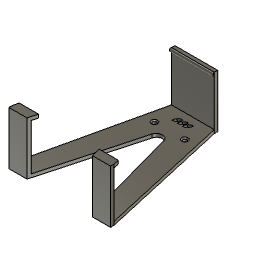
Sega Game Gear (Autodesk Fusion 360 design; units mm, degrees)
Autodesk Fusion 360 part; units mm, degrees
sketch "Top" plane through (0, 0, 0) normal (0, 0, 1) x (1, 0, 0)
  spline S0 degree 3 poles (50.664, -12.787) (49.4535, -14.1293) (47.9947, -14.8503) (47.407, -14.3973) knots 0 0 0 0 1 1 1 1
  spline S1 degree 3 poles (47.407, -14.3973) (46.8193, -13.9442) (47.3242, -12.4896) (48.5334, -11.1472) knots 1 1 1 1 2 2 2 2
  spline S2 degree 3 poles (48.5334, -11.1472) (49.7439, -9.8062) (51.2028, -9.0852) (51.7904, -9.5383) knots 2 2 2 2 3 3 3 3
  spline S3 degree 3 poles (51.7904, -9.5383) (52.3782, -9.9914) (51.8732, -11.446) (50.664, -12.787) knots 3 3 3 3 4 4 4 4
  spline S4 degree 3 poles (42.858, -14.3973) (42.2703, -13.9442) (42.7739, -12.4896) (43.9844, -11.1472) knots 0 0 0 0 1 1 1 1
  spline S5 degree 3 poles (43.9844, -11.1472) (45.1949, -9.8062) (46.6523, -9.0852) (47.2415, -9.5383) knots 1 1 1 1 2 2 2 2
  spline S6 degree 3 poles (47.2415, -9.5383) (47.8292, -9.9914) (47.3242, -11.446) (46.1137, -12.787) knots 2 2 2 2 3 3 3 3
  spline S7 degree 3 poles (46.1137, -12.787) (44.9032, -14.1293) (43.4458, -14.8503) (42.858, -14.3973) knots 3 3 3 3 4 4 4 4
  spline S8 degree 3 poles (38.2038, -14.4127) (37.6302, -13.9568) (38.1225, -12.4924) (39.3008, -11.143) knots 0 0 0 0 1 1 1 1
  spline S9 degree 3 poles (39.3008, -11.143) (40.4791, -9.7922) (41.8986, -9.0684) (42.4723, -9.5229) knots 1 1 1 1 2 2 2 2
  spline S10 degree 3 poles (42.4723, -9.5229) (43.0446, -9.9788) (42.5536, -11.4432) (41.374, -12.7926) knots 2 2 2 2 3 3 3 3
  spline S11 degree 3 poles (41.374, -12.7926) (40.1957, -14.1434) (38.7761, -14.8672) (38.2038, -14.4127) knots 3 3 3 3 4 4 4 4
  line L0 (64, -3) -> (64, 0)
  line L1 (64, 0) -> (26, 0)
  line L2 (26, 0) -> (26, -3)
  line L3 (26, -3) -> (0, -118)
  line L4 (0, -118) -> (0, -121)
  line L5 (0, -121) -> (16, -121)
  line L6 (16, -121) -> (39.812, -33.9631)
  spline S12 degree 3 poles (39.812, -33.9631) (41.2562, -28.684) (48.7438, -28.684) (50.188, -33.9631) knots 7 7 7 7 8 8 8 8
  line L7 (50.188, -33.9631) -> (74, -121)
  line L8 (74, -121) -> (90, -121)
  line L9 (90, -121) -> (90, -118)
  line L10 (90, -118) -> (64, -3)
extrude "Extrude1" add sketch "Top" along normal blind 57
sketch "RightSideCut" plane through (0, 0, 0) normal (1, 0, 0) x (0, 1, 0)
  line L0 (-121, 57) -> (-121, 47)
  line L1 (-121, 47) -> (-113, 47)
  line L2 (-113, 47) -> (-113, 44)
  line L3 (-113, 44) -> (-118, 44)
  line L4 (-118, 44) -> (-118, 3)
  line L5 (-118, 3) -> (-3, 3)
  line L6 (-3, 3) -> (-3, 44)
  spline S0 degree 3 poles (-3, 44) (-3.8284, 44) (-4.5, 44.6716) (-4.5, 46.3285) (-3.8284, 47) (-3, 47) knots 7 7 7 7 8 8 9 9 9 9
  line L7 (-3, 47) -> (0, 47)
  line L8 (0, 47) -> (0, 57)
  line L9 (0, 57) -> (-121, 57)
extrude "Extrude2" cut sketch "RightSideCut" along normal blind 90
hole "Hole1" at (31.5835, -23.65, 3) direction (0, 0, -1) diameter 3.5 depth 3 tip angle 118 countersink diameter 5.5 countersink angle 90
hole "Hole2" at (58.4162, -23.65, 3) direction (0, 0, -1) diameter 3.5 depth 3 tip angle 118 countersink diameter 5.5 countersink angle 90
